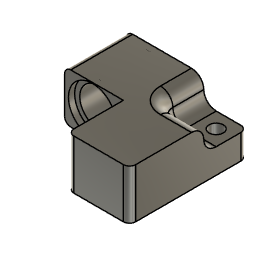
Board Bracket - Cube v1 (Autodesk Fusion 360 design; units mm, degrees)
Autodesk Fusion 360 part; units mm, degrees
note: some values were not read from the file. Chosen so that the rebuilt part matches the saved one: which face or edge a step refers to. Set by a fixed rule: which sketch regions a step uses.
sketch "Sketch1" plane through (0, 0, 0) normal (0, 0, 1) x (1, 0, 0)
  line L0 (15, 20) -> (0, 20)
  line L1 (0, 20) -> (0, 0)
  line L2 (0, 0) -> (8, 0)
  line L3 (8, 0) -> (8, 8)
  line L4 (8, 8) -> (15, 8)
  line L5 (15, 20) -> (15, 8)
  dimension "d2" = 20
  constraint horizontal L0
  constraint vertical L1
  constraint coincident L1.end L2.start
  constraint perpendicular L1 L2
  constraint perpendicular L4 L5
  measures "d2" distance of L1.end L0.end
extrude "Extrude1" add sketch "Sketch1" along normal blind 8
sketch "Sketch2" plane through (0, 0, 0) normal (0, -1, 0) x (1, 0, 0)
  line L0 (0, 0) -> (8, 0)
  line L1 (8, 0) -> (8, 8)
  line L2 (8, 8) -> (0, 8)
  line L3 (0, 8) -> (0, 0)
  line L4 (0, 8) -> (8, 0) construction
  line L5 (8, 8) -> (0, 0) construction
  circle A0 centre (4, 4) radius 3.875
  circle A1 centre (4, 4) radius 3.05
  dimension "d5" = 7.75
  dimension "d6" = 6.1
  constraint coincident L2.end L3.start
  constraint coincident L0.end L1.start
  constraint coincident L1.end L2.start
  constraint coincident L0.start L3.end
  constraint midpoint L5 A0.centre
  constraint concentric A0 A1
  measures "d5" diameter of A0
  measures "d6" diameter of A1
extrude "Extrude2" cut sketch "Sketch2" against normal blind 1 contours A0
extrude "Extrude3" cut 1 faces at (4.846, 0, 2.8674) along direction (0, 1, 0) blind 10
sketch "Sketch3" plane through (0, 0, 8) normal (0, 0, 1) x (-1, 0, 0)
  line L0 (0, -20) -> (0, 0)
  line L1 (0, 0) -> (-8, 0)
  line L2 (-15, -8) -> (-15, -20)
  line L3 (-15, -20) -> (0, -20)
  line L4 (-15, -20) -> (-6, -20)
  line L5 (-15, -11) -> (-15, -20)
  line L6 (0, 0) -> (0, -10)
  line L7 (0, -10) -> (-8, -10)
  line L8 (-8, -10) -> (-8, 0)
  line L9 (-8, 0) -> (0, 0)
  line L10 (0, 0) -> (0, -10)
  line L11 (-8, 0) -> (-8, -8)
  line L12 (-8, -8) -> (-15, -8)
  constraint horizontal L4
  constraint vertical L5
  constraint coincident L2.end L3.start
  constraint coincident L0.end L1.start
  constraint midpoint L0 L6.end
  constraint horizontal L7
  constraint vertical L8
  constraint horizontal L9
  constraint vertical L10
  constraint coincident L1.end L8.end
extrude "Extrude4" cut sketch "Sketch3" against normal blind 4.5 contours L0 L2 L3 L4 L5 L7 L8 L12
sketch "Sketch4" plane through (0, 10, 0) normal (0, -1, 0) x (1, 0, 0)
  line L0 (7.0087, 3.5) -> (0.9913, 3.5)
  arc A0 (0.9913, 3.5) -> (7.0087, 3.5) centre (4, 4) ccw
sketch "Sketch5" plane through (0, 10, 0) normal (0, -1, 0) x (1, 0, 0)
  circle A0 centre (4, 4) radius 3.875
  dimension "d15" = 7.75
  measures "d15" diameter of A0
extrude "Extrude5" cut sketch "Sketch5" along normal blind 1
extrude "Extrude6" add 1 faces at (12.6667, 8, 2.3333) along direction (0, -1, 0) blind 18
extrude "Extrude7" cut 1 faces at (10, 20, 1.1667) along direction (0, -1, 0) blind 10
extrude "Extrude8" add 1 faces at (12.6667, 0, 3.5) along direction (0, 0, 1) blind 4.5
extrude "Extrude9" cut 1 faces at (8, -3.3333, 2.6667) along direction (1, 0, 0) blind 1
extrude "Extrude10" add 1 faces at (15, 3.3333, 2.6667) along direction (1, 0, 0) blind 2
extrude "Extrude11" add 1 faces at (17, 3.3333, 2.6667) along direction (1, 0, 0) blind 2
sketch "Sketch6" plane through (0, 0, 8) normal (0, 0, 1) x (-1, 0, 0)
  line L0 (-9, 0) -> (-9, 10)
  line L1 (-9, 10) -> (-19, 10)
  line L2 (-19, 10) -> (-19, -10)
  line L3 (-19, -10) -> (0, -10)
  line L4 (0, -10) -> (0, 0)
  line L5 (0, 0) -> (-9, 0)
  line L6 (-19, -10) -> (-14, -10)
  line L7 (-14, -10) -> (-14, -5)
  line L8 (-14, -5) -> (-19, -5)
  line L9 (-19, -5) -> (-19, -10)
  line L10 (-19, -10) -> (-12, -10)
  line L11 (-12, -10) -> (-12, -3)
  line L12 (-12, -3) -> (-19, -3)
  line L13 (-19, -3) -> (-19, -10)
  line L14 (-19, -5) -> (-14, -10) construction
  line L15 (-14, -5) -> (-19, -10) construction
  circle A0 centre (-16.5, -7.5) radius 1.15
  dimension "d30" = 5
  dimension "d31" = 5
  dimension "d32" = 7
  dimension "d33" = 7
  dimension "d43" = 2.3
  constraint horizontal L6
  constraint vertical L7
  constraint horizontal L8
  constraint vertical L9
  constraint coincident L2.end L3.start
  constraint horizontal L10
  constraint vertical L11
  constraint horizontal L12
  constraint vertical L13
  constraint midpoint L14 A0.centre
  measures "d30" distance of L2.end L6.end
  measures "d31" distance of L2.end L8.end
  measures "d32" distance of L2.end L10.end
  measures "d33" distance of L2.end L12.end
  measures "d43" diameter of A0
extrude "Extrude12" cut sketch "Sketch6" against normal blind 4 contours L2 L3 L6 L7 L8 L9 L10 L13 | A0
extrude "Extrude13" cut sketch "Sketch6" against normal blind 4 contours L2 L3 L7 L8 L10 L11 L12 L13
move_face "OffsetFaces1" offset -1 1 faces at (15.6667, -10, 2.6667)
fillet "Fillet2" radius 2 3 edges at (15.5, 3, 4) (12, 3, 6) (12, 6.5, 4)
fillet "Fillet3" radius 1 3 edges at (19, 10, 2) (19, -9, 4) (9, -9, 4)
extrude "Extrude14" cut sketch "Sketch6" against normal blind 18 contours A0
fillet "Fillet4" radius 2 3 edges at (16.5, 3, 8) (12.5858, 3.5858, 8) (12, 7.5, 8)
move_face "OffsetFaces2" offset 0.5 1 faces at (0, 6.6667, 2.6667)
fillet "Fillet5" radius 1 2 edges at (-0.5, 5, 8) (-0.5, 5, 0)
